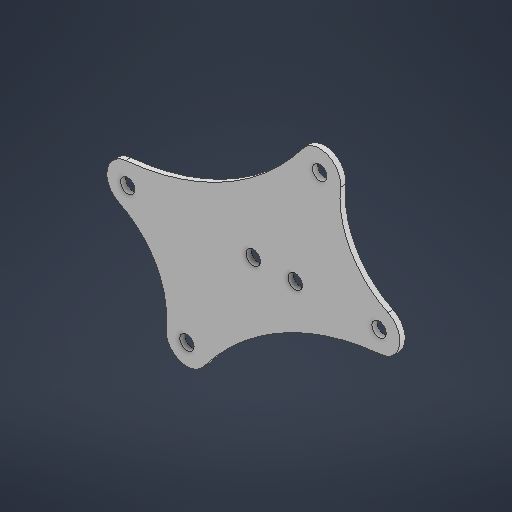
# Autodesk Inventor part: Side Poly
Saved by Autodesk Inventor 2025.1 (Build 291241000, 241)
## iProperties
Created: 2025-01-09
Part Number: Side Poly
Material: Generic
Document SubType Name: Modeling
Designer: Derek Chen
Density: 1 g/cm^3
Appearance: Default
Author: Derek Chen
Autodesk Inventor part; units mm, degrees
ref_plane "YZ Plane" through (0, 0, 0) normal (1, 0, 0) x (0, 1, 0)
ref_plane "XZ Plane" through (0, 0, 0) normal (0, 1, 0) x (-1, 0, 0)
ref_plane "XY Plane" through (0, 0, 0) normal (0, 0, 1) x (1, 0, 0)
sketch "Sketch1" plane through (0, 0, 0) normal (0, 0, 1) x (1, 0, 0)
  circle A0 centre (-74.1769, -5.2291) radius 2.1844
  circle A1 centre (-36.0455, -5.0199) radius 2.1844
  circle A2 centre (-112.2444, -5.4371) radius 2.1844
  circle A3 centre (-94.297, -37.5832) radius 2.1844
  circle A4 centre (-54.0568, 27.1251) radius 2.1844
  arc A5 (-35.4519, -11.3421) -> (-89.2225, -41.4005) centre (-28.3285, -87.2084) ccw
  arc A6 (-100.6091, -36.8907) -> (-114.967, -11.1738) centre (-125.8576, -34.1206) ccw
  arc A7 (-112.8432, 0.8846) -> (-59.1316, 30.942) centre (-120.0293, 76.745) ccw
  arc A8 (-47.7441, 26.4385) -> (-33.335, 0.7226) centre (-22.4929, 23.6923) ccw
  arc A9 (-35.4519, -11.3421) -> (-33.335, 0.7226) centre (-36.0455, -5.0199) ccw
  arc A10 (-100.6091, -36.8907) -> (-89.2225, -41.4005) centre (-94.297, -37.5832) ccw
  arc A11 (-112.8432, 0.8846) -> (-114.967, -11.1738) centre (-112.2444, -5.4371) ccw
  arc A12 (-47.7441, 26.4385) -> (-59.1316, 30.942) centre (-54.0568, 27.1251) ccw
  circle A13 centre (-61.4451, -5.159) radius 2.1844
  point P0 (-47.7441, 26.4385)
  dimension "d6" = 25.4
  dimension "d7" = 25.4
  dimension "d8" = 76.2
  dimension "d9" = 76.2
  constraints: 16 point on circle, 14 centre point, 3 coincident
  measures "d6" radius of A6
  measures "d7" radius of A8
  measures "d8" radius of A7
  measures "d9" radius of A5
extrude "Extrusion2" add sketch "Sketch1" along normal blind 1.5875
body "Solid2"
